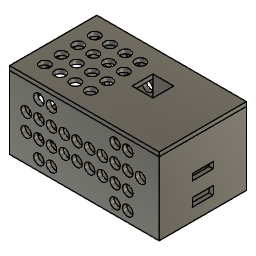
Shell (Autodesk Fusion 360 design; units mm, degrees)
Autodesk Fusion 360 part; units mm, degrees
sketch "Sketch2" plane through (0, 0, 0) normal (0, 0, 1) x (1, 0, 0)
  line L0 (-33, 21) -> (39, 21)
  line L1 (39, 21) -> (39, -21)
  line L2 (39, -21) -> (-33, -21)
  line L3 (-33, -21) -> (-33, 21)
  line L4 (50, 0) -> (-55, 0) construction
  circle A0 centre (34, -13) radius 2.5
  circle A1 centre (-18, -13) radius 2.5
  circle A2 centre (-18, 13) radius 2.5
  circle A3 centre (34, 13) radius 2.5
  dimension "d2" = 42
  dimension "d3" = 72
  dimension "d4" = 5
  dimension "d5" = 13
  dimension "d6" = 5
  dimension "d7" = 5
  dimension "d8" = 13
  dimension "d9" = 52
  dimension "d35" = 21
  constraint horizontal L0
  constraint vertical L1
  constraint horizontal L2
  constraint vertical L3
  constraint horizontal L4
  constraint symmetric L4 A0 A3
  constraint symmetric L4 A1 A2
  measures "d2" distance of L0.start L2.end
  measures "d3" distance of L0.start L0.end
  measures "d4" diameter of A0
  measures "d5" distance of L4 A0.centre
  measures "d6" distance of L1 A0.centre
  measures "d7" diameter of A1
  measures "d8" distance of L4 A1.centre
  measures "d9" distance of A0.centre A1.centre
  measures "d35" distance of L0 L4
extrude "Extrude1" add sketch "Sketch2" along normal blind 35 contours L0 L1 L2 L3 | A0 | A1 | A2 | A3 makes body 1
shell "Shell1" thickness 2 removed faces 1 at (-9, 7, 35) on bodies 1
extrude "Extrude2" add sketch "Sketch2" along normal blind 9.5 contours A0 | A1 | A2 | A3 bodies 1
sketch "Sketch3" plane through (0, 0, 9.5) normal (0, 0, 1) x (-1, 0, 0)
  circle A0 centre (18, -13) radius 1.25
  circle A1 centre (18, 13) radius 1.25
  circle A2 centre (-34, -13) radius 1.25
  circle A3 centre (-34, 13) radius 1.25
  circle A4 centre (-34, 13) radius 2.5
  dimension "d15" = 2.5
  dimension "d16" = 2.5
  dimension "d17" = 2.5
  dimension "d18" = 2.5
  measures "d15" diameter of A0
  measures "d16" diameter of A1
  measures "d17" diameter of A2
  measures "d18" diameter of A3
extrude "Extrude3" add sketch "Sketch3" along normal blind 2 contours A0 | A1 | A2 | A3 bodies 1
sketch "Sketch4" plane through (0, 0, 35) normal (0, 0, 1) x (-1, 0, 0)
  line L0 (33, 21) -> (-39, 21)
  line L1 (-39, 21) -> (-39, -21)
  line L2 (-39, -21) -> (33, -21)
  line L3 (33, -21) -> (33, 21)
  line L4 (31, 19) -> (31, -19)
  line L5 (31, -19) -> (-37, -19)
  line L6 (-37, -19) -> (-37, 19)
  line L7 (-37, 19) -> (31, 19)
sketch "Sketch5" plane through (39, 0, 0) normal (1, 0, 0) x (0, 1, 0)
  line L0 (-21, 0) -> (21, 0)
  line L1 (21, 0) -> (21, 35)
  line L2 (21, 35) -> (-21, 35)
  line L3 (-21, 35) -> (-21, 0)
  line L4 (-5, 10) -> (5, 10)
  line L5 (5, 10) -> (5, 6)
  line L6 (5, 6) -> (-5, 6)
  line L7 (-5, 6) -> (-5, 10)
  line L8 (21, 0) -> (-21, 0)
  dimension "d23" = 6
  dimension "d24" = 10
  dimension "d25" = 4
  constraint horizontal L4
  constraint vertical L5
  constraint horizontal L6
  constraint vertical L7
  measures "d23" distance of L6 L8
  measures "d24" distance of L4.start L4.end
  measures "d25" distance of L4.start L6.end
extrude "Extrude4" cut sketch "Sketch5" against normal blind 2 contours L4 L5 L6 L7 bodies 1
sketch "Sketch6" plane through (-33, 0, 0) normal (-1, 0, 0) x (0, -1, 0)
  line L0 (-21, 0) -> (21, 0)
  line L1 (21, 0) -> (21, 35)
  line L2 (21, 35) -> (-21, 35)
  line L3 (-21, 35) -> (-21, 0)
  line L4 (-13.5, 10) -> (13.5, 10)
  line L5 (13.5, 10) -> (13.5, 26)
  line L6 (13.5, 26) -> (-13.5, 26)
  line L7 (-13.5, 26) -> (-13.5, 10)
  line L8 (-13.5, 26) -> (13.5, 10) construction
  line L9 (-13.5, 10) -> (13.5, 26) construction
  line L10 (21, 0) -> (-21, 0) construction
  dimension "d28" = 27
  dimension "d29" = 16
  dimension "d30" = 10
  constraint horizontal L4
  constraint vertical L5
  constraint horizontal L6
  constraint vertical L7
  measures "d28" distance of L4.start L4.end
  measures "d29" distance of L4.start L6.end
  measures "d30" distance of L4 L10
extrude "Extrude5" cut sketch "Sketch6" against normal blind 2 contours L4 L5 L6 L7 bodies 1
sketch "Sketch9" plane through (0, 0, 2) normal (0, 0, 1) x (-1, 0, 0)
  circle A0 centre (-34, -13) radius 2.5
  circle A1 centre (18, -13) radius 2.5
  circle A2 centre (-34, 13) radius 2.5
  circle A3 centre (18, 13) radius 2.5
  line L0 (31, 19) -> (-37, 19)
  line L1 (-37, 19) -> (-37, -19)
  line L2 (-37, -19) -> (31, -19)
  line L3 (31, -19) -> (31, 19)
  line L4 (25.25, -19) -> (27.75, -19)
  line L5 (27.75, -19) -> (27.75, -9)
  line L6 (27.75, -9) -> (25.25, -9)
  line L7 (25.25, -9) -> (25.25, -19)
  line L8 (-50, 0) -> (55, 0)
  line L9 (27.75, 19) -> (27.75, 9)
  line L10 (25.25, 19) -> (27.75, 19)
  line L11 (25.25, 9) -> (25.25, 19)
  line L12 (27.75, 9) -> (25.25, 9)
  dimension "d40" = 2.5
  dimension "d41" = 10
  dimension "d42" = 3.25
  constraint horizontal L4
  constraint vertical L5
  constraint horizontal L6
  constraint vertical L7
  constraint coincident L2 L4.start
  constraint symmetric L4.start L8 L10.start
  constraint symmetric L4.end L8 L9.start
  constraint symmetric L5.end L8 L9.end
  constraint symmetric L6.end L8 L11.start
  measures "d40" distance of L4.start L4.end
  measures "d41" distance of L4.start L6.end
  measures "d42" distance of L3 L5
extrude "Extrude6" add sketch "Sketch9" along normal blind 4 contours L0 L9 L10 L11 L12 | L2 L4 L5 L6 L7 bodies 1
sketch "Sketch10" plane through (0, -21, 0) normal (0, -1, 0) x (1, 0, 0)
  line L0 (-33, 0) -> (39, 0)
  line L1 (39, 0) -> (39, 35)
  line L2 (39, 35) -> (-33, 35)
  line L3 (-33, 35) -> (-33, 0)
  circle A0 centre (-25, 30) radius 2.5
  circle A1 centre (-18.8889, 30) radius 2.5
  circle A2 centre (-12.7778, 30) radius 2.5
  circle A3 centre (-6.6667, 30) radius 2.5
  circle A4 centre (-0.5556, 30) radius 2.5
  circle A5 centre (5.5556, 30) radius 2.5
  circle A6 centre (11.6667, 30) radius 2.5
  circle A7 centre (17.7778, 30) radius 2.5
  circle A8 centre (23.8889, 30) radius 2.5
  circle A9 centre (30, 30) radius 2.5
  circle A10 centre (-25, 21.6667) radius 2.5
  circle A11 centre (-18.8889, 21.6667) radius 2.5
  circle A12 centre (-12.7778, 21.6667) radius 2.5
  circle A13 centre (-6.6667, 21.6667) radius 2.5
  circle A14 centre (-0.5556, 21.6667) radius 2.5
  circle A15 centre (5.5556, 21.6667) radius 2.5
  circle A16 centre (11.6667, 21.6667) radius 2.5
  circle A17 centre (17.7778, 21.6667) radius 2.5
  circle A18 centre (23.8889, 21.6667) radius 2.5
  circle A19 centre (30, 21.6667) radius 2.5
  circle A20 centre (-25, 13.3333) radius 2.5
  circle A21 centre (-18.8889, 13.3333) radius 2.5
  circle A22 centre (-12.7778, 13.3333) radius 2.5
  circle A23 centre (-6.6667, 13.3333) radius 2.5
  circle A24 centre (-0.5556, 13.3333) radius 2.5
  circle A25 centre (5.5556, 13.3333) radius 2.5
  circle A26 centre (11.6667, 13.3333) radius 2.5
  circle A27 centre (17.7778, 13.3333) radius 2.5
  circle A28 centre (23.8889, 13.3333) radius 2.5
  circle A29 centre (30, 13.3333) radius 2.5
  circle A30 centre (-25, 5) radius 2.5
  circle A31 centre (-18.8889, 5) radius 2.5
  circle A32 centre (-12.7778, 5) radius 2.5
  circle A33 centre (-6.6667, 5) radius 2.5
  circle A34 centre (-0.5556, 5) radius 2.5
  circle A35 centre (5.5556, 5) radius 2.5
  circle A36 centre (11.6667, 5) radius 2.5
  circle A37 centre (17.7778, 5) radius 2.5
  circle A38 centre (23.8889, 5) radius 2.5
  circle A39 centre (30, 5) radius 2.5
  dimension "d45" = 5
  dimension "d48" = 55
  dimension "d49" = -25
  measures "d45" diameter of A0
extrude "Extrude7" cut sketch "Sketch10" against normal blind 2 contours A1 | A2 | A7 | A8 | A10 | A11 | A12 | A13 | A14 | A15 | A16 | A17 | A18 | A19 | A20 | A21 | A22 | A23 | A24 | A25 | A26 | A27 | A28 | A31 | A32 | A37 | A38 bodies 1
sketch "Sketch11" plane through (0, 21, 0) normal (0, 1, 0) x (-1, 0, 0)
  line L0 (-39, 0) -> (33, 0)
  line L1 (33, 0) -> (33, 35)
  line L2 (33, 35) -> (-39, 35)
  line L3 (-39, 35) -> (-39, 0)
  circle A0 centre (-30, 30) radius 2.5
  circle A1 centre (-23.8889, 30) radius 2.5
  circle A2 centre (-17.7778, 30) radius 2.5
  circle A3 centre (-11.6667, 30) radius 2.5
  circle A4 centre (-5.5556, 30) radius 2.5
  circle A5 centre (0.5556, 30) radius 2.5
  circle A6 centre (6.6667, 30) radius 2.5
  circle A7 centre (12.7778, 30) radius 2.5
  circle A8 centre (18.8889, 30) radius 2.5
  circle A9 centre (25, 30) radius 2.5
  circle A10 centre (-30, 21.6667) radius 2.5
  circle A11 centre (-23.8889, 21.6667) radius 2.5
  circle A12 centre (-17.7778, 21.6667) radius 2.5
  circle A13 centre (-11.6667, 21.6667) radius 2.5
  circle A14 centre (-5.5556, 21.6667) radius 2.5
  circle A15 centre (0.5556, 21.6667) radius 2.5
  circle A16 centre (6.6667, 21.6667) radius 2.5
  circle A17 centre (12.7778, 21.6667) radius 2.5
  circle A18 centre (18.8889, 21.6667) radius 2.5
  circle A19 centre (25, 21.6667) radius 2.5
  circle A20 centre (-30, 13.3333) radius 2.5
  circle A21 centre (-23.8889, 13.3333) radius 2.5
  circle A22 centre (-17.7778, 13.3333) radius 2.5
  circle A23 centre (-11.6667, 13.3333) radius 2.5
  circle A24 centre (-5.5556, 13.3333) radius 2.5
  circle A25 centre (0.5556, 13.3333) radius 2.5
  circle A26 centre (6.6667, 13.3333) radius 2.5
  circle A27 centre (12.7778, 13.3333) radius 2.5
  circle A28 centre (18.8889, 13.3333) radius 2.5
  circle A29 centre (25, 13.3333) radius 2.5
  circle A30 centre (-30, 5) radius 2.5
  circle A31 centre (-23.8889, 5) radius 2.5
  circle A32 centre (-17.7778, 5) radius 2.5
  circle A33 centre (-11.6667, 5) radius 2.5
  circle A34 centre (-5.5556, 5) radius 2.5
  circle A35 centre (0.5556, 5) radius 2.5
  circle A36 centre (6.6667, 5) radius 2.5
  circle A37 centre (12.7778, 5) radius 2.5
  circle A38 centre (18.8889, 5) radius 2.5
  circle A39 centre (25, 5) radius 2.5
  dimension "d52" = 5
  dimension "d55" = 55
  dimension "d56" = -25
  measures "d52" diameter of A0
extrude "Extrude8" cut sketch "Sketch11" against normal blind 2 contours A1 | A2 | A7 | A8 | A10 | A11 | A12 | A13 | A14 | A15 | A16 | A17 | A18 | A19 | A20 | A21 | A22 | A23 | A24 | A25 | A26 | A27 | A28 | A29 | A31 | A32 | A37 | A38 bodies 1
sketch "Sketch12" plane through (39, 0, 0) normal (1, 0, 0) x (0, 1, 0)
  line L0 (5, 10) -> (5, 6)
  line L1 (5, 6) -> (-5, 6)
  line L2 (-5, 6) -> (-5, 10)
  line L3 (-5, 10) -> (5, 10)
  line L4 (-21, 0) -> (21, 0)
  line L5 (21, 0) -> (21, 35)
  line L6 (21, 35) -> (-21, 35)
  line L7 (-21, 35) -> (-21, 0)
  line L8 (-5, 20) -> (5, 20)
  line L9 (5, 20) -> (5, 17)
  line L10 (5, 17) -> (-5, 17)
  line L11 (-5, 17) -> (-5, 20)
  dimension "d59" = 10
  dimension "d60" = 3
  dimension "d61" = 15
  constraint horizontal L8
  constraint vertical L9
  constraint horizontal L10
  constraint vertical L11
  measures "d59" distance of L8.start L8.end
  measures "d60" distance of L8.start L10.end
  measures "d61" distance of L6 L8
extrude "Extrude9" cut sketch "Sketch12" against normal blind 2 contours L8 L9 L10 L11 bodies 1
sketch "Sketch1" plane through (0, 0, 35) normal (0, 0, 1) x (-1, 0, 0) in component "Case Top"
  line L0 (33, 21) -> (-39, 21)
  line L1 (-39, 21) -> (-39, -21)
  line L2 (-39, -21) -> (33, -21)
  line L3 (33, -21) -> (33, 21)
  line L4 (33, -21) -> (-39, -21)
  line L5 (-39, -21) -> (-39, 21)
  line L6 (-39, 21) -> (33, 21)
  line L7 (33, 21) -> (33, -21)
  constraint horizontal L4
  constraint vertical L5
  constraint horizontal L6
  constraint vertical L7
  constraint coincident L0.end L1.start
  constraint coincident L2.end L3.start
extrude "Extrude1'" add sketch "Sketch1" along normal blind 2 separate body makes body 2 in component "Case Top"
sketch "Sketch2 (2)" plane through (0, 0, 35) normal (0, 0, -1) x (1, 0, 0) in component "Case Top"
  line L0 (39, 21) -> (-33, 21)
  line L1 (-33, 21) -> (-33, -21)
  line L2 (-33, -21) -> (39, -21)
  line L3 (39, -21) -> (39, 21)
sketch "Sketch4 (2)" plane through (0, 0, 35) normal (0, 0, -1) x (1, 0, 0) in component "Case Top"
  line L0 (-31, -19) -> (37, -19)
  line L1 (37, -19) -> (37, 19)
  line L2 (37, 19) -> (-31, 19)
  line L3 (-31, 19) -> (-31, -19)
  constraint horizontal L0
  constraint vertical L1
  constraint horizontal L2
  constraint vertical L3
extrude "Extrude2'" add sketch "Sketch4 (2)" along normal blind 2 bodies 2 in component "Case Top"
shell "Shell1'" thickness 2 removed faces 1 at (-8.3333, 6.3333, 33) on bodies 2 in component "Case Top"
sketch "Sketch5 (2)" plane through (0, 0, 35) normal (0, 0, -1) x (1, 0, 0) in component "Case Top"
  line L0 (-47.9853, 0) -> (47.0147, 0) construction
  line L1 (-31.0003, 14) -> (-31.0003, 17)
  line L2 (-31.0003, -17) -> (-25.25, -17)
  line L3 (-25.25, -17) -> (-25.25, -14)
  line L4 (-25.25, -14) -> (-31.0003, -14)
  line L5 (-31.0003, -14) -> (-31.0003, -17)
  line L6 (-27.75, -14) -> (-27.75, 14)
  line L7 (-27.75, 14) -> (-25.25, 14)
  line L8 (-25.25, 14) -> (-25.25, -14)
  line L9 (-31, 19) -> (-31, -19)
  line L10 (-25.25, 14) -> (-25.25, 17)
  line L11 (-31.0003, 14) -> (-27.75, 14)
  line L12 (-25.25, 17) -> (-31.0003, 17)
  dimension "d69" = 14
  dimension "d71" = 3.25
  dimension "d72" = 2.5
  constraint horizontal L0
  constraint vertical L6
  constraint horizontal L7
  constraint vertical L8
  constraint perpendicular L6 L11
  constraint perpendicular L1 L12
  measures "d69" distance of L0 L4
  measures "d71" distance of L6 L9
  measures "d72" distance of L6 L8
extrude "Extrude3'" add sketch "Sketch5 (2)" along normal blind 10 contours L1 L7 L9 L10 L11 L12 | L2 L3 L4 L5 L9 | L4 L6 L7 L8 bodies 2 in component "Case Top"
sketch "Sketch14" plane through (0, 0, 25) normal (0, 0, -1) x (1, 0, 0)
  line L0 (-25.25, -17) -> (-25.25, 17)
  line L1 (-25.25, 17) -> (-31, 17)
  line L2 (-31, 17) -> (-31, 14)
  line L3 (-31, 14) -> (-27.75, 14)
  line L4 (-27.75, 14) -> (-27.75, -14)
  line L5 (-27.75, -14) -> (-31, -14)
  line L6 (-31, -14) -> (-31, -17)
  line L7 (-31, -17) -> (-25.25, -17)
sketch "Sketch6 (2)" plane through (0, 0, 25) normal (0, 0, -1) x (1, 0, 0) in component "Case Top"
  line L0 (-25.25, -17) -> (-25.25, 17)
  line L1 (-25.25, 17) -> (-31, 17)
  line L2 (-31, 17) -> (-31, 14)
  line L3 (-31, 14) -> (-27.75, 14)
  line L4 (-27.75, 14) -> (-27.75, -14)
  line L5 (-27.75, -14) -> (-31, -14)
  line L6 (-31, -14) -> (-31, -17)
  line L7 (-31, -17) -> (-25.25, -17)
  line L8 (-27.75, 10) -> (-25.25, 10)
  line L9 (-25.25, 10) -> (-25.25, -10)
  line L10 (-25.25, -10) -> (-27.75, -10)
  line L11 (-27.75, -10) -> (-27.75, 10)
extrude "Extrude4'" cut sketch "Sketch6 (2)" against normal blind 10 contours L0 L4 L8 L9 L10 L11 bodies 2 in component "Case Top"
sketch "Sketch7" plane through (0, 0, 35) normal (0, 0, -1) x (1, 0, 0) in component "Case Top"
  line L0 (-25.25, 17) -> (-25.25, 10)
  line L1 (-25.25, 10) -> (-27.75, 10)
  line L2 (-27.75, 10) -> (-27.75, 14)
  line L3 (-27.75, 14) -> (-29, 14)
  line L4 (-29, 14) -> (-29, -14)
  line L5 (-29, -14) -> (-27.75, -14)
  line L6 (-27.75, -14) -> (-27.75, -10)
  line L7 (-27.75, -10) -> (-25.25, -10)
  line L8 (-25.25, -10) -> (-25.25, -17)
  line L9 (-25.25, -17) -> (35, -17)
  line L10 (35, -17) -> (35, 17)
  line L11 (35, 17) -> (-25.25, 17)
  line L12 (-5, 0) -> (-5, -10)
  line L13 (-5, -10) -> (35, -10)
  line L14 (35, -10) -> (35, 0)
  line L15 (35, 0) -> (35, 10)
  line L16 (35, 10) -> (-5, 10)
  line L17 (-5, 10) -> (-5, 0)
  line L18 (5, 0) -> (15, 0)
  line L19 (15, 0) -> (15, -10)
  line L20 (15, -10) -> (5, -10)
  line L21 (5, -10) -> (5, 0)
  dimension "d78" = 40
  dimension "d81" = 10
  dimension "d82" = 10
  dimension "d83" = 10
  dimension "d84" = 20
  constraint horizontal L13
  constraint midpoint L10 L14.end
  constraint vertical L15
  constraint horizontal L16
  constraint vertical L17
  constraint horizontal L18
  constraint vertical L19
  constraint horizontal L20
  constraint vertical L21
  measures "d78" distance of L14.end L12.start
  measures "d81" distance of L12.start L16.end
  measures "d82" distance of L18.start L18.end
  measures "d83" distance of L18.start L20.end
  measures "d84" distance of L14 L19
extrude "Extrude5'" cut sketch "Sketch7" against normal blind 6 contours L13 L18 L19 L20 L21 bodies 2 in component "Case Top"
sketch "Sketch8" plane through (0, 0, 35) normal (0, 0, -1) x (1, 0, 0) in component "Case Top"
  line L0 (15, 0) -> (15, -10)
  line L1 (15, -10) -> (5, -10)
  line L2 (5, -10) -> (5, 0)
  line L3 (5, 0) -> (15, 0)
  line L4 (-25.25, 17) -> (-25.25, 10)
  line L5 (-25.25, 10) -> (-27.75, 10)
  line L6 (-27.75, 10) -> (-27.75, 14)
  line L7 (-27.75, 14) -> (-29, 14)
  line L8 (-29, 14) -> (-29, -14)
  line L9 (-29, -14) -> (-27.75, -14)
  line L10 (-27.75, -14) -> (-27.75, -10)
  line L11 (-27.75, -10) -> (-25.25, -10)
  line L12 (-25.25, -10) -> (-25.25, -17)
  line L13 (-25.25, -17) -> (35, -17)
  line L14 (35, -17) -> (35, 17)
  line L15 (35, 17) -> (-25.25, 17)
  line L16 (5, -10) -> (15, -10)
  line L17 (15, -10) -> (15, -12)
  line L18 (15, -12) -> (5, -12)
  line L19 (5, -12) -> (5, -10)
  line L20 (15, 12) -> (5, 12)
  line L21 (15, 10) -> (15, 12)
  line L22 (5, 10) -> (15, 10)
  line L23 (5, 12) -> (5, 10)
  dimension "d87" = 10
  dimension "d88" = 2
  constraint horizontal L16
  constraint vertical L17
  constraint horizontal L18
  constraint vertical L19
  constraint coincident L1.end L2.start
  constraint symmetric L3 L1.end L22.start
  constraint symmetric L3 L0.end L21.start
  constraint symmetric L3 L17.end L20.start
  constraint symmetric L3 L18.end L20.end
  measures "d87" distance of L1.end L0.end
  measures "d88" distance of L1.end L18.end
extrude "Extrude6'" add sketch "Sketch8" along normal blind 12 contours L1 L16 L17 L18 L19 bodies 2 in component "Case Top"
extrude "Extrude7'" add sketch "Sketch8" along normal blind 12 contours L20 L21 L22 L23 bodies 2 in component "Case Top"
sketch "Sketch9 (2)" plane through (0, -10, 0) normal (0, 1, 0) x (-1, 0, 0) in component "Case Top"
  line L0 (-5, 35) -> (-15, 35)
  line L1 (-15, 35) -> (-15, 23)
  line L2 (-15, 23) -> (-5, 23)
  line L3 (-5, 23) -> (-5, 35)
  line L4 (-15, 23) -> (-5, 23)
  line L5 (-5, 23) -> (-5, 25)
  line L6 (-5, 25) -> (-15, 25)
  line L7 (-15, 25) -> (-15, 23)
  dimension "d93" = 10
  dimension "d94" = 2
  constraint horizontal L4
  constraint vertical L5
  constraint horizontal L6
  constraint vertical L7
  constraint coincident L1.end L2.start
  measures "d93" distance of L1.end L2.end
  measures "d94" distance of L1.end L6.end
extrude "Extrude8'" add sketch "Sketch9 (2)" along normal blind 20 contours L1 L2 L3 L4 L5 L6 L7 bodies 2 in component "Case Top"
sketch "Sketch10 (2)" plane through (0, 0, 37) normal (0, 0, 1) x (-1, 0, 0) in component "Case Top"
  line L0 (-15, -10) -> (-15, 0)
  line L1 (-15, 0) -> (-5, 0)
  line L2 (-5, 0) -> (-5, -10)
  line L3 (-5, -10) -> (-15, -10)
  line L4 (33, 21) -> (-39, 21)
  line L5 (-39, 21) -> (-39, -21)
  line L6 (-39, -21) -> (33, -21)
  line L7 (33, -21) -> (33, 21)
  line L8 (28, -15) -> (0, -15)
  line L9 (0, -15) -> (0, 15)
  line L10 (0, 15) -> (28, 15)
  line L11 (28, 15) -> (28, -15)
  circle A0 centre (25, -12) radius 2.5
  circle A1 centre (17.6667, -12) radius 2.5
  circle A2 centre (10.3333, -12) radius 2.5
  circle A3 centre (3, -12) radius 2.5
  circle A4 centre (25, -4) radius 2.5
  circle A5 centre (17.6667, -4) radius 2.5
  circle A6 centre (10.3333, -4) radius 2.5
  circle A7 centre (3, -4) radius 2.5
  circle A8 centre (25, 4) radius 2.5
  circle A9 centre (17.6667, 4) radius 2.5
  circle A10 centre (10.3333, 4) radius 2.5
  circle A11 centre (3, 4) radius 2.5
  circle A12 centre (25, 12) radius 2.5
  circle A13 centre (17.6667, 12) radius 2.5
  circle A14 centre (10.3333, 12) radius 2.5
  circle A15 centre (3, 12) radius 2.5
  dimension "d97" = 28
  dimension "d98" = 30
  dimension "d99" = 6
  dimension "d100" = 5
  dimension "d101" = 3
  dimension "d102" = 3
  dimension "d105" = -22
  dimension "d106" = 24
  constraint horizontal L8
  constraint vertical L9
  constraint horizontal L10
  constraint vertical L11
  measures "d97" distance of L8.start L8.end
  measures "d98" distance of L8.start L10.end
  measures "d99" distance of L6 L8
  measures "d100" diameter of A0
  measures "d101" distance of L8 A0.centre
  measures "d102" distance of L11 A0.centre
extrude "Extrude9'" cut sketch "Sketch10 (2)" against normal blind 2 contours A0 | A1 | A2 | A3 | A4 | A5 | A6 | A7 | A8 | A9 | A10 | A11 | A12 | A13 | A14 | A15 bodies 2 in component "Case Top"
sketch "Sketch13" plane through (0, 0, 35) normal (0, 0, -1) x (1, 0, 0)
component "Case Top" placed x (1, 0, 0) y (0, 1, 0) z (0, 0, 1) at (0, 0, 0)
equation "d2 = 40 mm + Shell"
equation "d3 = 70 mm + Shell"
equation "d6 = 3 mm + Shell"
equation "Shell = 2 mm"
equation "d11 = Height"
equation "d13 = 7.5 mm + Shell"
equation "Height = 35 mm"
equation "d22 = Shell"
equation "d26 = -Shell"
equation "d31 = -Shell"
equation "d64 = Shell"
equation "d66 = Shell"
equation "d68 = Shell"
equation "d88 = Shell"
equation "d89 = 10 mm + Shell"
equation "d91 = 10 mm + Shell"
